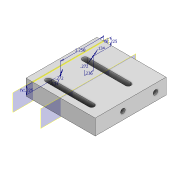
# Autodesk Inventor part: driven wheel mount to xrail
Saved by Autodesk Inventor 2020 (Build 240168000, 168)
## iProperties
Created: 2020-01-25
Part Number: driven wheel mount to xrail
Material: Generic
Document SubType Name: Modeling
Designer: ball
Density: 1 g/cm^3
Appearance: Default
Author: ball
Autodesk Inventor part; units mm, degrees
ref_plane "YZ Plane" through (0, 0, 0) normal (1, 0, 0) x (0, 1, 0)
ref_plane "XZ Plane" through (0, 0, 0) normal (0, 1, 0) x (-1, 0, 0)
ref_plane "XY Plane" through (0, 0, 0) normal (0, 0, 1) x (1, 0, 0)
sketch "Sketch1" plane through (0, 0, 0) normal (0, 1, 0) x (-1, 0, 0)
  line L0 (-25.4, 20.32) -> (-25.4, -31.75)
  line L1 (-25.4, -31.75) -> (25.4, -31.75)
  line L2 (25.4, -31.75) -> (25.4, 20.32)
  line L3 (25.4, 31.75) -> (-25.4, -31.75) construction
  line L4 (-25.4, 31.75) -> (25.4, -31.75) construction
  line L5 (15.875, 13.4747) -> (-15.875, 13.4747) construction
  line L6 (15.875, 15.5067) -> (-15.875, 15.5067)
  line L7 (-15.875, 11.4427) -> (15.875, 11.4427)
  arc A0 (15.875, 11.4427) -> (15.875, 15.5067) centre (15.875, 13.4747) ccw
  arc A1 (-15.875, 15.5067) -> (-15.875, 11.4427) centre (-15.875, 13.4747) ccw
  line L8 (-15.875, -13.4747) -> (15.875, -13.4747) construction
  line L9 (-15.875, -15.5067) -> (15.875, -15.5067)
  line L10 (15.875, -11.4427) -> (-15.875, -11.4427)
  arc A2 (-15.875, -11.4427) -> (-15.875, -15.5067) centre (-15.875, -13.4747) ccw
  arc A3 (15.875, -15.5067) -> (15.875, -11.4427) centre (15.875, -13.4747) ccw
  line L11 (25.4, 20.32) -> (-25.4, 20.32)
  point P0 (0, 0)
  point P1 (0, 13.4747)
  point P2 (0, -13.4747)
  dimension "d0" = 50.8
  dimension "d2" = 26.9494
  dimension "d3" = 13.4747
  dimension "d4" = 26.9494
  dimension "d6" = 9.525
  dimension "d7" = 9.525
  dimension "d10" = 4.064
  dimension "d11" = 9.525
  dimension "d12" = 4.064
  dimension "d49" = 6.8453
  constraints: 28 end point, 8 point on circle, 8 tangent, 4 centre point, 4 midpoint, 3 parallel, 2 horizontal, 1 perpendicular
  measures "d0" distance of L1.end L0.end
  measures "d2" distance of L5.start L8.end
  measures "d3" vertical distance of point (0, 0) L8.end
  measures "d4" distance of L8.start L5.end
  measures "d6" distance from line of L2 L5.start
  measures "d7" distance from line of L2 L8.end
  measures "d10" diameter of A1
  measures "d11" distance from line of L0 L5.end
  measures "d12" diameter of A3
  measures "d49" distance from line of L11 L5.start
extrude "Extrusion1" add sketch "Sketch1" along normal blind 11.43
sketch "Sketch3" plane through (0, 0, 0) normal (0, -1, 0) x (1, 0, 0)
  arc A0 (-15.875, -11.4427) -> (-15.875, -15.5067) centre (-15.875, -13.4747) ccw projected
  arc A1 (15.875, -15.5067) -> (15.875, -11.4427) centre (15.875, -13.4747) ccw projected
  line L0 (-15.875, -13.4747) -> (15.875, -13.4747) construction
  line L1 (-15.875, -17.9197) -> (15.875, -17.9197)
  line L2 (15.875, -9.0297) -> (-15.875, -9.0297)
  arc A2 (-15.875, -9.0297) -> (-15.875, -17.9197) centre (-15.875, -13.4747) ccw
  arc A3 (15.875, -17.9197) -> (15.875, -9.0297) centre (15.875, -13.4747) ccw
  arc A4 (-15.875, 15.5067) -> (-15.875, 11.4427) centre (-15.875, 13.4747) ccw projected
  arc A5 (15.875, 11.4427) -> (15.875, 15.5067) centre (15.875, 13.4747) ccw projected
  line L3 (-15.875, 13.4747) -> (15.875, 13.4747) construction
  line L4 (-15.875, 9.0297) -> (15.875, 9.0297)
  line L5 (15.875, 17.9197) -> (-15.875, 17.9197)
  arc A6 (-15.875, 17.9197) -> (-15.875, 9.0297) centre (-15.875, 13.4747) ccw
  arc A7 (15.875, 9.0297) -> (15.875, 17.9197) centre (15.875, 13.4747) ccw
  point P0 (0, 0)
  point P1 (0, -13.4747)
  point P2 (0, 13.4747)
  dimension "d19" = 8.89
  dimension "d20" = 8.89
  constraints: 16 end point, 8 point on circle, 8 tangent, 4 centre point, 2 horizontal, 2 midpoint, 2 parallel
  measures "d19" diameter of A3
  measures "d20" diameter of A7
extrude "Extrusion3" cut sketch "Sketch3" against normal blind 5.9436
ref_plane "Work Plane2" through (-20.4, 0, -31.75) normal (-1, 0, 0) x (0, 0, 1)
sketch "Sketch5" plane through (-20.4, 0, -31.75) normal (-1, 0, 0) x (0, 0, 1)
  circle A0 centre (31.75, 5.715) radius 3.45 construction
  line L0 (52.07, 0) -> (0, 0) projected
  line L1 (52.07, 11.43) -> (0, 11.43) projected
  line L2 (0, 0) -> (0, 11.43) projected
  line L3 (28.7622, 0) -> (28.7622, 7.44)
  line L4 (28.7622, 7.44) -> (31.75, 9.165)
  line L5 (31.75, 9.165) -> (34.7378, 7.44)
  line L6 (34.7378, 7.44) -> (34.7378, 0)
  line L7 (28.7622, 0) -> (34.7378, 0)
  line L8 (13.8303, 0) -> (13.8303, 5.9436) construction
  line L9 (49.6697, 0) -> (49.6697, 5.9436) construction
  circle A1 centre (7.8403, 5.715) radius 3.45 construction
  line L10 (4.8525, 0) -> (4.8525, 7.44)
  line L11 (4.8525, 7.44) -> (7.8403, 9.165)
  line L12 (7.8403, 9.165) -> (10.8281, 7.44)
  line L13 (10.8281, 7.44) -> (10.8281, 0)
  line L14 (4.8525, 0) -> (10.8281, 0)
  circle A2 centre (7.8403, 5.715) radius 1.7
  circle A3 centre (31.75, 5.715) radius 1.7
  point P0 (31.75, 0)
  dimension "d24" = 6.9
  dimension "d26" = 5.715
  dimension "d29" = 6.9
  dimension "d31" = 5.99
  dimension "d33" = 5.715
  dimension "d37" = 3.4
  dimension "d38" = 3.4
  dimension "d48" = 31.75
  constraints: 20 end point, 4 centre point, 3 coincident, 2 point on line, 6 other
  measures "d24" diameter of A0
  measures "d26" distance from line of L1 A0.centre
  measures "d29" diameter of A1
  measures "d31" distance from line of L8 A1.centre
  measures "d33" distance from line of L1 A1.centre
  measures "d37" diameter of A2
  measures "d38" diameter of A3
  measures "d48" distance from line of A0.centre L2
extrude "Extrusion4" cut sketch "Sketch5" along normal blind 2.8 contours L0 L10 L11 L12 L13 | L0 L3 L4 L5 L6 | A2 | A3
sketch "Sketch6" plane through (-25.4, 0, -31.75) normal (-1, 0, 0) x (0, 0, 1)
  circle A0 centre (7.8403, 5.715) radius 1.7
  circle A1 centre (31.75, 5.715) radius 1.7
  line L0 (13.8303, 0) -> (13.8303, 5.9436) projected
  line L1 (63.5, 0) -> (63.5, 11.43) projected
  line L2 (49.6697, 0) -> (49.6697, 5.9436) projected
  point P0 (31.75, 0)
  dimension "d40" = 3.4
  dimension "d41" = 3.4
  dimension "d43" = 5.99
  constraints: 2 centre point
  measures "d40" diameter of A0
  measures "d41" diameter of A1
  measures "d43" distance from line of A0.centre L0
extrude "Extrusion5" cut sketch "Sketch6" against normal blind 6
ref_plane "Work Plane3" through (0, 0, -31.75) normal (-1, 0, 0) x (0, 0, 1)
mirror "Mirror1" about plane through (0, 0, -31.75) normal (-1, 0, 0) of "Extrusion4"
mirror "Mirror2" about plane through (0, 0, -31.75) normal (-1, 0, 0) of "Extrusion5"
sketch "Sketch7" plane through (0, 0, 0) normal (0, -1, 0) x (1, 0, 0)
  point P0 (0, 0)
equation "\"d3\" = 0.5 * d2"
equation "\"d4\" = d2"
equation "\"d26\" = 0.5 * d25"
equation "\"d33\" = d26"
equation "\"d43\" = d31"
equation "\"d25\" = 11.43"
body "Solid1"
